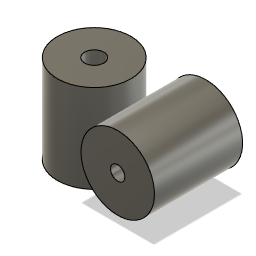
ShoulderAxle_1 v16 (Autodesk Fusion 360 design; units mm, degrees)
Autodesk Fusion 360 part; units mm, degrees
note: some values were not read from the file. Set by a fixed rule: which sketch regions a step uses.
cylinder "CylinderPrimitive1" add diameter 25 height 30 placed x (1, 0, 0) y (0, 0, -1) z (0, 1, 0) at (0, 0, 0) makes body 1
ref_plane "WorkPlane1" through (10, 0, 0) normal (1, 0, 0) x (0, 1, 0)
sketch "Sketch2" plane through (10, 0, 0) normal (1, 0, 0) x (0, 0, -1)
  circle A0 centre (0, 15) radius 6
extrude "Extrude1" add sketch "Sketch2" along normal blind -3 and the other way blind -10 bodies 1
sketch "Sketch3" plane through (0, 0, 0) normal (0, 0, 1) x (1, 0, 0)
  circle A0 centre (23, 15) radius 12.5
  dimension "d27" = 25
  measures "d27" diameter of A0
extrude "Extrude2" add sketch "Sketch3" along normal mid plane 30 bodies 1
sketch "Sketch4" plane through (0, 30, 0) normal (0, 1, 0) x (-1, 0, 0)
  circle A0 centre (0, 0) radius 12.5
  circle A1 centre (0, 0) radius 3.25
  dimension "d10" = 6.5
  constraint concentric A0 A1
  measures "d10" diameter of A1
extrude "Extrude3" cut sketch "Sketch4" against normal blind 16 contours A1 bodies 1
sketch "Sketch5" plane through (0, 0, -15) normal (0, 0, -1) x (-1, 0, 0)
  circle A0 centre (-23, 15) radius 3.25
  circle A1 centre (-23, 15) radius 12.5
  dimension "d13" = 6.5
  measures "d13" diameter of A0
extrude "Extrude4" cut sketch "Sketch5" against normal blind 16 contours A0 bodies 1
copy_body "Body->Comp1" bodies 1 removing the originals makes body 2 in component "Component"
sketch "Sketch8" plane through (0, 0, 1) normal (0, 0, -1) x (-1, 0, 0)
  circle A0 centre (-23, 15) radius 3.25
  line L0 (-17.9794, 13.9286) -> (-20.013, 13.7191)
  line L1 (-17.9794, 13.9286) -> (-20.1526, 13.4333)
  point P0 (-17, 11.75)
  constraint coincident A0 L0.end
  constraint coincident A0 L1.end
extrude "Extrude3'" add sketch "Sketch8" along normal blind 7 contours A0 L0 L1 bodies 2 in component "Component"
sketch "Sketch9" plane through (0, 14, 0) normal (0, 1, 0) x (-1, 0, 0)
  circle A0 centre (0, 0) radius 3.25
  line L0 (2.75, 0) -> (2.75, -1.7321)
  line L1 (2.75, 0) -> (2.75, 1.7321)
  constraint coincident A0 L0.end
  constraint coincident A0 L1.end
extrude "Extrude4'" add sketch "Sketch9" against normal blind 0.5 contours A0 L0 L1 picked at (3.0727, 0.1517) bodies 2 in component "Component"
sketch "Sketch6" plane through (0, 0, 0) normal (0, -1, 0) x (1, 0, 0)
  circle A0 centre (0, 0) radius 12.5
  circle A1 centre (0, 0) radius 2.45
  dimension "d16" = 4.9
  constraint concentric A0 A1
  measures "d16" diameter of A1
extrude "Extrude1'" cut sketch "Sketch6" against normal blind 15 contours A1 bodies 2 in component "Component"
sketch "Sketch7" plane through (0, 0, 15) normal (0, 0, 1) x (1, 0, 0)
  circle A0 centre (23, 15) radius 2.45
  circle A1 centre (23, 15) radius 12.5
  dimension "d19" = 4.9
  measures "d19" diameter of A0
extrude "Extrude2'" cut sketch "Sketch7" against normal blind 20 contours A0 bodies 2 in component "Component"
component "Component" placed x (1, 0, 0) y (0, 1, 0) z (0, 0, 1) at (0, 0, 0)
